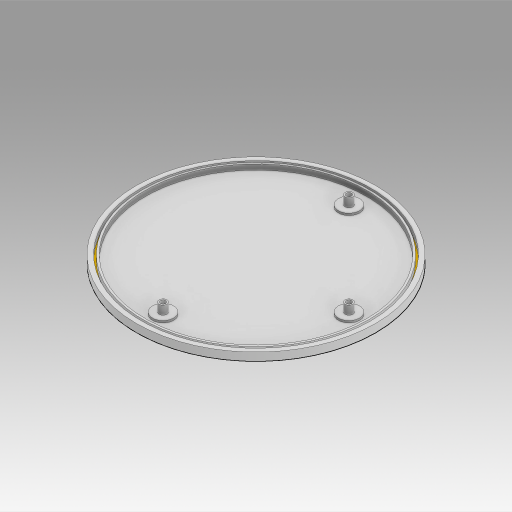
# Autodesk Inventor part: ROUNDBOTTOMCOVER
Saved by Autodesk Inventor 2023 (Build 270158000, 158)
## iProperties
Created: 2025-09-17
Part Number: ROUNDBOTTOMCOVER
Material: Generic
Document SubType Name: Modeling
Designer: NELLY NDUNG'U
Density: 1 g/cm^3
Appearance: Default
Author: NELLY NDUNG'U
Autodesk Inventor part; units mm, degrees
ref_plane "YZ Plane" through (0, 0, 0) normal (1, 0, 0) x (0, 1, 0)
ref_plane "XZ Plane" through (0, 0, 0) normal (0, 1, 0) x (-1, 0, 0)
ref_plane "XY Plane" through (0, 0, 0) normal (0, 0, 1) x (1, 0, 0)
sketch "Sketch1" plane through (0, 0, 0) normal (0, 1, 0) x (-1, 0, 0)
  circle A0 centre (0, 0) radius 45
  dimension "d0" = 90
  constraints: 1 centre point, 1 coincident
  measures "d0" diameter of A0
extrude "Extrusion1" add sketch "Sketch1" along normal blind 3
sketch "Sketch2" plane through (0, 3, 0) normal (0, 1, 0) x (1, 0, 0)
  circle A0 centre (0, 0) radius 45 projected
  circle A1 centre (0, 0) radius 42.5
  circle A2 centre (0, 0) radius 43.25
  circle A3 centre (0, 0) radius 41.75
  dimension "d3" = 2.5
  dimension "d4" = 0.75
  dimension "d5" = 0.75
  constraints: 3 centre point
  measures "d3" radial gap between concentric circles of A0 A1
  measures "d4" radial gap between concentric circles of A1 A2
  measures "d5" radial gap between concentric circles of A1 A3
extrude "Extrusion2" cut sketch "Sketch2" against normal blind 2 contours A3
extrude "Extrusion3" cut sketch "Sketch2" against normal blind 2 contours A2
sketch "Sketch3" plane through (0, 1, 0) normal (0, 1, 0) x (1, 0, 0)
  circle A0 centre (0, 0) radius 40 construction
  line L0 (-40, 0) -> (40, 0) construction
  line L1 (0, 40) -> (0, -40) construction
  circle A1 centre (0, 35) radius 1.5
  circle A2 centre (35, 0) radius 1.5
  circle A3 centre (0, -35) radius 1.5
  circle A4 centre (0, 35) radius 4
  circle A5 centre (35, 0) radius 4
  circle A6 centre (0, -35) radius 4
  dimension "d10" = 80
  dimension "d12" = 3
  dimension "d13" = 3
  dimension "d14" = 5
  dimension "d15" = 5
  dimension "d17" = 3
  dimension "d18" = 5
  dimension "d19" = 2.5
  dimension "d20" = 2.5
  dimension "d21" = 2.5
  constraints: 7 centre point, 4 end point, 4 point on circle, 3 point on line, 1 coincident, 1 horizontal, 1 perpendicular
  measures "d10" diameter of A0
  measures "d12" diameter of A1
  measures "d13" diameter of A2
  measures "d14" distance of A1.centre L1.start
  measures "d15" distance of L0.end A2.centre
  measures "d17" diameter of A3
  measures "d18" distance of L1.end A3.centre
  measures "d19" radial gap between concentric circles of A1 A4
  measures "d20" radial gap between concentric circles of A2 A5
  measures "d21" radial gap between concentric circles of A3 A6
extrude "Extrusion4" add sketch "Sketch3" along normal blind 0.75
extrude "Extrusion6" add sketch "Sketch3" along normal blind 4 contours A1 | A2 | A3
sketch "Sketch5" plane through (35, 5, 0) normal (0, 1, 0) x (1, 0, 0)
  circle A0 centre (0, 0) radius 4 projected
  circle A1 centre (-35, -35) radius 4 projected
  circle A2 centre (-35, 35) radius 4 projected
  circle A3 centre (-35, 35) radius 1.5 projected
  circle A4 centre (-35, 35) radius 1
  circle A5 centre (0, 0) radius 1.5 projected
  circle A6 centre (0, 0) radius 1
  circle A7 centre (-35, -35) radius 1.5 projected
  circle A8 centre (-35, -35) radius 1
  point P0 (-35, 0)
  dimension "d30" = 0.5
  dimension "d31" = 0.5
  dimension "d32" = 0.5
  constraints: 3 centre point
  measures "d30" radial gap between concentric circles of A3 A4
  measures "d31" radial gap between concentric circles of A5 A6
  measures "d32" radial gap between concentric circles of A7 A8
extrude "Extrusion7" cut sketch "Sketch5" against normal through all contours A4 | A6 | A8
body "Solid1"
